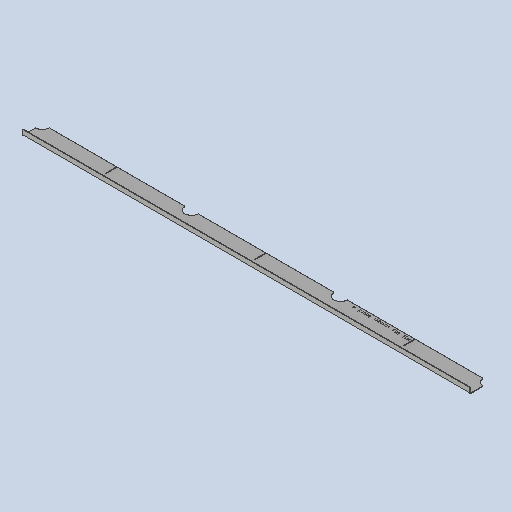
# Autodesk Inventor part: MSC 063 stringer board #
Saved by Autodesk Inventor 2025 (Build 290162010, 162A)
## iProperties
Created: 2024-04-28
Part Number: MSC 063 stringer board #
Material: Stainless Steel
Document SubType Name: Sheet Metal
Designer: pokla
Density: 8 g/cm^3
Sheet Metal Rule: AISI304 2mm Die16
Appearance: Default
Flat Pattern Width: 150 cm
Flat Pattern Length: 8.3565 cm
Flat Pattern Area: 1253.48 cm^2
Sheet Metal Width: 1500,000 mm
Sheet Metal Length: 83,565 mm
Sheet Metal Area: 125347,506 mm^2
Stock Number: МОО 063 стрингер борт #
Author: admin
Autodesk Inventor part; units mm, degrees
ref_plane "YZ Plane" through (0, 0, 0) normal (1, 0, 0) x (0, 1, 0)
ref_plane "XZ Plane" through (0, 0, 0) normal (0, 1, 0) x (-1, 0, 0)
ref_plane "XY Plane" through (0, 0, 0) normal (0, 0, 1) x (1, 0, 0)
sketch "Sketch1" plane through (0, 0, 0) normal (0, 0, 1) x (1, 0, 0)
  line L0 (-750, 67.363) -> (750, 67.363)
  line L1 (750, 67.363) -> (750, 0)
  line L2 (750, 0) -> (-750, 0)
  line L3 (-750, 0) -> (-750, 67.363)
  point P0 (0, 0)
  point P1 (0, 0)
  dimension "d0" = 1500
  dimension "d1" = 67.363
  measures "d0" distance of L1.end L2.end
  measures "d1" distance of L0.end L1.end
extrude "Plate1" add sketch "Sketch1" along normal blind 2
sketch "Sketch2" plane through (750, 2, 0) normal (0, -1, 0) x (1, 0, 0)
  line L0 (-1500, 0) -> (0, 0)
  line L1 (0, 0) -> (0, 20)
  line L2 (0, 20) -> (-1500, 20)
  line L3 (-1500, 20) -> (-1500, 0)
  constraints: 6 end point, 1 horizontal, 1 perpendicular, 1 vertical
edge flange "Flange1" height 20 angle 90 thickness 2 bend radius 2.75 thickness toward (0, -1, 0) relief round relief width 2 relief depth 1 edges at (0, 0, 2) wall of the first edge with corners at (-750, 2, 0) (750, 2, 0) (750, 2, 20) (-750, 2, 20)
bend "Bend1"
corner "Corner1"
sketch "Sketch5" plane through (0, 0, 0) normal (0, 0, -1) x (-1, 0, 0)
  line L0 (750, 67.363) -> (-750, 67.363) projected
  line L1 (-1, 30) -> (-1, 67.363)
  line L2 (750, 0) -> (-750, 0) projected
  line L3 (-1, 30) -> (1, 30)
  line L4 (1, 30) -> (1, 67.363)
  point P0 (0, 0)
  point P1 (0, 30)
  point P2 (0, 0)
  dimension "d27" = 2
  dimension "d28" = 30
  constraints: 6 end point, 2 midpoint, 2 point on line, 1 horizontal, 1 parallel, 1 perpendicular, 1 vertical alignment
  measures "d27" distance of L1.start L3.end
  measures "d28" distance of point (0, 0) point (0, 30)
extrude "Extrusion1" cut sketch "Sketch5" against normal through all
pattern_linear "Rectangular Pattern1" count 3 spacing 500 along (1, 0, 0) of "Extrusion1" first direction both ways yes
sketch "Sketch6" plane through (0, 0, 0) normal (0, 0, -1) x (-1, 0, 0)
  line L0 (-750, 67.363) -> (-750, 4.75) projected
  circle A0 centre (-750, 67.363) radius 22.5
  line L1 (-750, 67.363) -> (750, 67.363) projected
  line L2 (-1, 30) -> (-1, 67.363) projected
  line L3 (-499, 67.363) -> (-499, 30) projected
  line L4 (-1, 30) -> (-499, 30) construction
  circle A1 centre (-250, 67.363) radius 22.5
  point P0 (0, 0)
  point P1 (-727.5, 67.363)
  point P2 (-750, 44.863)
  point P3 (-250, 30)
  dimension "d24" = 45
  constraints: 2 centre point, 2 end point, 1 equal radius, 1 midpoint, 1 perpendicular, 1 point on line, 1 vertical alignment
  measures "d24" diameter of A0
extrude "Extrusion2" cut sketch "Sketch6" along normal mid plane 30 contours L1 A0 L0 | A1 L1 | L1 A1 picked at (-748.3311, 52.551)
mirror "Mirror1" about plane through (0, 0, 0) normal (1, 0, 0) of "Extrusion2"
sketch "Sketch7" plane through (0, 0, 2) normal (0, 0, 1) x (1, 0, 0)
  arc A0 (-750, 44.863) -> (-727.5, 67.363) centre (-750, 67.363) ccw projected
  line L0 (-750, 4.75) -> (-750, 44.863) projected
  line L1 (-750, 4.75) -> (750, 4.75) projected
  line L2 (750, 44.863) -> (750, 4.75) projected
  arc A1 (727.5, 67.363) -> (750, 44.863) centre (750, 67.363) ccw projected
  line L3 (501, 67.363) -> (727.5, 67.363) projected
  line L4 (501, 67.363) -> (501, 30) projected
  line L5 (501, 30) -> (499, 30) projected
  line L6 (499, 30) -> (499, 67.363) projected
  line L7 (1, 67.363) -> (227.5, 67.363) projected
  line L8 (1, 67.363) -> (1, 30) projected
  line L9 (1, 30) -> (-1, 30) projected
  line L10 (-1, 30) -> (-1, 67.363) projected
  line L11 (-499, 67.363) -> (-272.5, 67.363) projected
  line L12 (-499, 67.363) -> (-499, 30) projected
  line L13 (-499, 30) -> (-501, 30) projected
  line L14 (-501, 30) -> (-501, 67.363) projected
  line L15 (-727.5, 67.363) -> (-501, 67.363) projected
  line L16 (650, 4.75) -> (650, 67.363) construction
  line L17 (-750, 4.75) -> (750, 4.75) projected
  circle A2 centre (650, 36.0565) radius 5
  line L18 (272.5, 67.363) -> (499, 67.363) projected
  arc A3 (227.5, 67.363) -> (272.5, 67.363) centre (250, 67.363) ccw projected
  line L19 (-227.5, 67.363) -> (-1, 67.363) projected
  arc A4 (-272.5, 67.363) -> (-227.5, 67.363) centre (-250, 67.363) ccw projected
  point P0 (0, 0)
  dimension "d29" = 100
  dimension "d30" = 10
  constraints: 2 end point, 2 point on line, 1 centre point, 1 coincident, 1 midpoint, 1 perpendicular
  measures "d29" distance from line of L2 L16.end
  measures "d30" diameter of A2
extrude "Extrusion3" [suppressed]
mirror "Mirror2" [suppressed]
sketch "Sketch8" plane through (0, 0, 2) normal (0, 0, 1) x (1, 0, 0)
  line L0 (494, 62.363) -> (494, 50.363) construction
  line L1 (494, 50.363) -> (294, 50.363) construction
  line L2 (294, 50.363) -> (294, 62.363) construction
  line L3 (294, 62.363) -> (494, 62.363) construction
  line L4 (501, 67.363) -> (727.5, 67.363) projected
  line L5 (272.5, 67.363) -> (499, 67.363) projected
  point P0 (0, 0)
  dimension "d33" = 200
  dimension "d34" = 12
  dimension "d37" = 5
  dimension "d38" = 5
  constraints: 2 other
  measures "d33" distance of L0.end L1.end
  measures "d34" distance of L1.end L2.end
  measures "d37" distance between parallel lines of L5 L3
  measures "d38" distance from line of L0 L5.end
mark "Mark2"
equation "\"d28\" = Стрингер_глубина_паза"
equation "\"d1\" = Стрингер_3"
equation "\"d27\" = d18"
equation "\"d2\" = Thickness"
equation "\"d3\" = BendReliefWidth"
equation "\"d4\" = BendReliefDepth"
equation "\"d5\" = MinimumRemnant"
equation "\"d6\" = TransitionRadius"
equation "\"d9\" = BendRadius"
equation "\"d10\" = CornerReliefSize"
equation "\"d11\" = GapSize"
equation "\"d12\" = JacobiRadiusSize"
equation "\"BendReliefWidth\" = Thickness"
equation "\"BendReliefDepth\" = 0.5 * Thickness"
equation "\"CornerReliefSize\" = 4 * Thickness"
equation "\"MinimumRemnant\" = 2 * Thickness"
equation "\"TransitionRadius\" = BendRadius"
equation "\"JacobiRadiusSize\" = BendRadius"
equation "\"GapSize\" = Thickness"
equation "\"d18\" = Thickness"
equation "\"Стрингер_3\" = 67.363014"
equation "\"Thickness\" = 2"
equation "\"BendRadius\" = 2.75"
equation "\"Стрингер_глубина_паза\" = 30"
body "Solid1"
